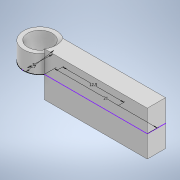
# Autodesk Inventor part: Part1
Saved by Autodesk Inventor 2022 (Build 260153000, 153)
## iProperties
Created: 2022-03-28
Part Number: Part1
Material: Generic
Document SubType Name: Modeling
Designer: Hajar
Density: 1 g/cm^3
Appearance: Default
Author: Hajar
Autodesk Inventor part; units mm, degrees
ref_plane "YZ Plane" through (0, 0, 0) normal (1, 0, 0) x (0, 1, 0)
ref_plane "XZ Plane" through (0, 0, 0) normal (0, 1, 0) x (-1, 0, 0)
ref_plane "XY Plane" through (0, 0, 0) normal (0, 0, 1) x (1, 0, 0)
sketch "Sketch1" plane through (0, 0, 0) normal (0, 1, 0) x (-1, 0, 0)
  circle A0 centre (0, 0) radius 2.5
  circle A1 centre (0, 0) radius 3.35
  line L0 (-3.35, 0) -> (-15.85, 0) construction
  line L1 (-2.7822, 1.866) -> (-23.7822, 1.866)
  line L2 (-2.7822, -1.866) -> (-23.7822, -1.866)
  line L3 (-23.7822, -1.866) -> (-23.7822, 1.866)
  point P0 (0.2218, 3.3427)
  point P1 (0.2218, -3.3427)
  dimension "d0" = 5
  dimension "d1" = 6.7
  dimension "d2" = 12.5
  dimension "d12" = 21
  constraints: 8 end point, 5 point on circle, 3 horizontal, 2 centre point, 2 coincident, 1 perpendicular
  measures "d0" diameter of A0
  measures "d1" diameter of A1
  measures "d2" distance of L0.start L0.end
  measures "d12" distance of L1.start L1.end
extrude "Extrusion1" add sketch "Sketch1" along normal blind 3.7 contours A1
extrude "Extrusion3" add sketch "Sketch1" along normal mid plane 9 contours A1 L2 L3 L1
body "Solid1"
